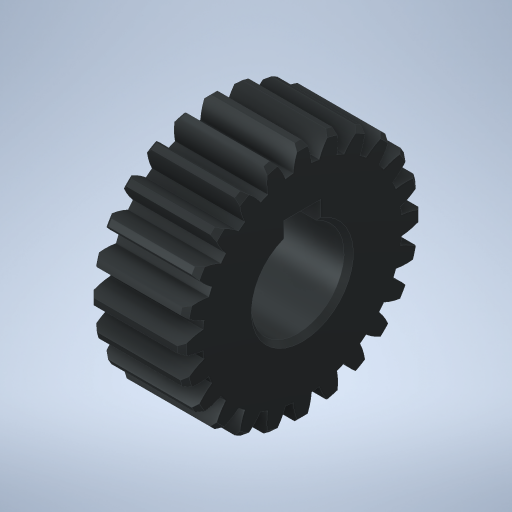
# Autodesk Inventor part: SSA1-24J10_On
Saved by Autodesk Inventor 2023 (Build 270158000, 158)
## iProperties
Category: PARTsolutions
Company: KHK
Created: 2023-07-21
Part Number: SSA1-24J10_On
Material: Iron, Cast
Catalog Web Link: www.cadenas.de
Description: Steel, Hubless Spur Gears (SSA)-
Vendor: KHK
Document SubType Name: Modeling
Designer: psAdmin
Manufacturer: KHK
Mass: 25.4574 g
Surface Area: 25.5099 cm^2
Volume: 3.56048 cm^3
Density: 7.15 g/cm^3
Appearance: Iron Gray
PSOL_IDENT_0: {$CADENAS_DATA/23d-libs/khk/spur_gears/steel_hubless_spur_gears_ssa.prj},198 {VTYP=3D},{NB=SSA1-24J1
PSOL_IDENT_1: 0_On},{LINA=SSA1-24J10},{NN=Steel, Hubless Spur Gears (SSA)},{DATE=06.10.2022 23:14:57},{GEOMDATE=26
PSOL_IDENT_2: .04.2021 06:49:50},{VERSION=},{LINEID=1180},{WBVAR=TOOTH,HT},{WBNUMERIC=}  {NB=SSA1-24J10_On},{LINA=
PSOL_IDENT_3: SSA1-24J10},{KT=DUMMY},{CN=SSA1-24J10},{CN1=SSA1-24J10},{A=10},{VER=1},{KW=4},{KD=1.8},{S=S5K},{SOLD=
PSOL_IDENT_4: S5K},{M=1},{MX=1.000},{Z=24},{B=0},{C=24.0},{D=26.0},{E=10},{F=0},{H=0},{I=0},{WMF=S5001.WMF},{N=0.5
PSOL_IDENT_5: },{L=0.5},{R=0},{L2=0},{VERS=0},{TOOTH=On},{HT=}
NB: SSA1-24J10_On
NN: Steel, Hubless Spur Gears (SSA)
NBSYN: $CN._$TOOTH.
LINA: SSA1-24J10
CATALOG: KHK
CN: SSA1-24J10
A: 10
KW: 4
KD: 1.8
S: S5K
M: 1
Z: 24
C: 24
D: 26
E: 10
TOOTH: On
HT: without
SUPPLIER: KHK
ARTICLENO: SSA1-24J10_On
BOMINFO: SSA1-24J10
CREATOR: CADENAS GmbH
Title: SSA1-24J10
Author: Cadenas PARTsolutions
Autodesk Inventor part; units mm, degrees
ref_plane "YZ Plane" through (0, 0, 0) normal (1, 0, 0) x (0, 1, 0)
ref_plane "XZ Plane" through (0, 0, 0) normal (0, 1, 0) x (-1, 0, 0)
ref_plane "XY Plane" through (0, 0, 0) normal (0, 0, 1) x (1, 0, 0)
sketch "Sketch_1" plane through (0, 0, 0) normal (0, 0, 1) x (1, 0, 0)
  line L0 (10, 0) -> (0, 0)
  line L1 (0, 5.5) -> (0.5, 5)
  line L2 (0.5, 5) -> (9.5, 5)
  line L3 (9.5, 5) -> (10, 5.5)
  line L4 (10, 5.5) -> (10, 12.5)
  line L5 (10, 12.5) -> (9.5, 13)
  line L6 (9.5, 13) -> (0.5, 13)
  line L7 (0.5, 13) -> (0, 12.5)
  line L8 (0, 12.5) -> (0, 5.5)
  constraints: 18 end point
revolve "Revolution1" add sketch "Sketch_1" angle 360 about axis through (10, 0, 0) along (1, 0, 0)
sketch "Sketch_6" plane through (0, 0, 0) normal (1, 0, 0) x (0, 1, 0)
  line L0 (0, 2) -> (0, -2)
  line L1 (0, -2) -> (6.8, -2)
  line L2 (6.8, -2) -> (6.8, 2)
  line L3 (6.8, 2) -> (0, 2)
  constraints: 8 end point
extrude "Extrusion1" cut sketch "Sketch_6" along normal blind 10
sketch "Sketch_7" plane through (0, 0, 0) normal (1, 0, 0) x (0, 1, 0)
  line L0 (26, 26) -> (-26, 26)
  line L1 (-26, 26) -> (-26, -26)
  line L2 (-26, -26) -> (26, -26)
  line L3 (26, -26) -> (26, 26)
  arc A0 (0.3403, 12.9955) -> (-0.3403, 12.9955) centre (0, 0) ccw
  arc A1 (-0.3403, 12.9955) -> (-0.9836, 10.7049) centre (4.9998, 10.2601) ccw
  arc A2 (-0.9836, 10.7049) -> (-1.8205, 10.5947) centre (0, 0) ccw
  arc A3 (-1.8205, 10.5947) -> (-3.0348, 12.6408) centre (-7.485, 8.6164) ccw
  arc A4 (-3.0348, 12.6408) -> (-3.6922, 12.4647) centre (0, 0) ccw
  arc A5 (-3.6922, 12.4647) -> (-3.7208, 10.0856) centre (2.174, 11.2045) ccw
  arc A6 (-3.7208, 10.0856) -> (-4.5006, 9.7625) centre (0, 0) ccw
  arc A7 (-4.5006, 9.7625) -> (-6.2031, 11.4246) centre (-9.46, 6.3856) ccw
  arc A8 (-6.2031, 11.4246) -> (-6.7925, 11.0843) centre (0, 0) ccw
  arc A9 (-6.7925, 11.0843) -> (-6.2043, 8.7789) centre (-0.8, 11.3854) ccw
  arc A10 (-6.2043, 8.7789) -> (-6.874, 8.265) centre (0, 0) ccw
  arc A11 (-6.874, 8.265) -> (-8.9486, 9.4299) centre (-10.7904, 3.7195) ccw
  arc A12 (-8.9486, 9.4299) -> (-9.4299, 8.9486) centre (0, 0) ccw
  arc A13 (-9.4299, 8.9486) -> (-8.265, 6.874) centre (-3.7195, 10.7904) ccw
  arc A14 (-8.265, 6.874) -> (-8.7789, 6.2043) centre (0, 0) ccw
  arc A15 (-8.7789, 6.2043) -> (-11.0843, 6.7925) centre (-11.3854, 0.8) ccw
  arc A16 (-11.0843, 6.7925) -> (-11.4246, 6.2031) centre (0, 0) ccw
  arc A17 (-11.4246, 6.2031) -> (-9.7625, 4.5006) centre (-6.3856, 9.46) ccw
  arc A18 (-9.7625, 4.5006) -> (-10.0856, 3.7208) centre (0, 0) ccw
  arc A19 (-10.0856, 3.7208) -> (-12.4647, 3.6922) centre (-11.2045, -2.174) ccw
  arc A20 (-12.4647, 3.6922) -> (-12.6408, 3.0348) centre (0, 0) ccw
  arc A21 (-12.6408, 3.0348) -> (-10.5947, 1.8205) centre (-8.6164, 7.485) ccw
  arc A22 (-10.5947, 1.8205) -> (-10.7049, 0.9836) centre (0, 0) ccw
  arc A23 (-10.7049, 0.9836) -> (-12.9955, 0.3403) centre (-10.2601, -4.9998) ccw
  arc A24 (-12.9955, 0.3403) -> (-12.9955, -0.3403) centre (0, 0) ccw
  arc A25 (-12.9955, -0.3403) -> (-10.7049, -0.9836) centre (-10.2601, 4.9998) ccw
  arc A26 (-10.7049, -0.9836) -> (-10.5947, -1.8205) centre (0, 0) ccw
  arc A27 (-10.5947, -1.8205) -> (-12.6408, -3.0348) centre (-8.6164, -7.485) ccw
  arc A28 (-12.6408, -3.0348) -> (-12.4647, -3.6922) centre (0, 0) ccw
  arc A29 (-12.4647, -3.6922) -> (-10.0856, -3.7208) centre (-11.2045, 2.174) ccw
  arc A30 (-10.0856, -3.7208) -> (-9.7625, -4.5006) centre (0, 0) ccw
  arc A31 (-9.7625, -4.5006) -> (-11.4246, -6.2031) centre (-6.3856, -9.46) ccw
  arc A32 (-11.4246, -6.2031) -> (-11.0843, -6.7925) centre (0, 0) ccw
  arc A33 (-11.0843, -6.7925) -> (-8.7789, -6.2043) centre (-11.3854, -0.8) ccw
  arc A34 (-8.7789, -6.2043) -> (-8.265, -6.874) centre (0, 0) ccw
  arc A35 (-8.265, -6.874) -> (-9.4299, -8.9486) centre (-3.7195, -10.7904) ccw
  arc A36 (-9.4299, -8.9486) -> (-8.9486, -9.4299) centre (0, 0) ccw
  arc A37 (-8.9486, -9.4299) -> (-6.874, -8.265) centre (-10.7904, -3.7195) ccw
  arc A38 (-6.874, -8.265) -> (-6.2043, -8.7789) centre (0, 0) ccw
  arc A39 (-6.2043, -8.7789) -> (-6.7925, -11.0843) centre (-0.8, -11.3854) ccw
  arc A40 (-6.7925, -11.0843) -> (-6.2031, -11.4246) centre (0, 0) ccw
  arc A41 (-6.2031, -11.4246) -> (-4.5006, -9.7625) centre (-9.46, -6.3856) ccw
  arc A42 (-4.5006, -9.7625) -> (-3.7208, -10.0856) centre (0, 0) ccw
  arc A43 (-3.7208, -10.0856) -> (-3.6922, -12.4647) centre (2.174, -11.2045) ccw
  arc A44 (-3.6922, -12.4647) -> (-3.0348, -12.6408) centre (0, 0) ccw
  arc A45 (-3.0348, -12.6408) -> (-1.8205, -10.5947) centre (-7.485, -8.6164) ccw
  arc A46 (-1.8205, -10.5947) -> (-0.9836, -10.7049) centre (0, 0) ccw
  arc A47 (-0.9836, -10.7049) -> (-0.3403, -12.9955) centre (4.9998, -10.2601) ccw
  arc A48 (-0.3403, -12.9955) -> (0.3403, -12.9955) centre (0, 0) ccw
  arc A49 (0.3403, -12.9955) -> (0.9836, -10.7049) centre (-4.9998, -10.2601) ccw
  arc A50 (0.9836, -10.7049) -> (1.8205, -10.5947) centre (0, 0) ccw
  arc A51 (1.8205, -10.5947) -> (3.0348, -12.6408) centre (7.485, -8.6164) ccw
  arc A52 (3.0348, -12.6408) -> (3.6922, -12.4647) centre (0, 0) ccw
  arc A53 (3.6922, -12.4647) -> (3.7208, -10.0856) centre (-2.174, -11.2045) ccw
  arc A54 (3.7208, -10.0856) -> (4.5006, -9.7625) centre (0, 0) ccw
  arc A55 (4.5006, -9.7625) -> (6.2031, -11.4246) centre (9.46, -6.3856) ccw
  arc A56 (6.2031, -11.4246) -> (6.7925, -11.0843) centre (0, 0) ccw
  arc A57 (6.7925, -11.0843) -> (6.2043, -8.7789) centre (0.8, -11.3854) ccw
  arc A58 (6.2043, -8.7789) -> (6.874, -8.265) centre (0, 0) ccw
  arc A59 (6.874, -8.265) -> (8.9486, -9.4299) centre (10.7904, -3.7195) ccw
  arc A60 (8.9486, -9.4299) -> (9.4299, -8.9486) centre (0, 0) ccw
  arc A61 (9.4299, -8.9486) -> (8.265, -6.874) centre (3.7195, -10.7904) ccw
  arc A62 (8.265, -6.874) -> (8.7789, -6.2043) centre (0, 0) ccw
  arc A63 (8.7789, -6.2043) -> (11.0843, -6.7925) centre (11.3854, -0.8) ccw
  arc A64 (11.0843, -6.7925) -> (11.4246, -6.2031) centre (0, 0) ccw
  arc A65 (11.4246, -6.2031) -> (9.7625, -4.5006) centre (6.3856, -9.46) ccw
  arc A66 (9.7625, -4.5006) -> (10.0856, -3.7208) centre (0, 0) ccw
  arc A67 (10.0856, -3.7208) -> (12.4647, -3.6922) centre (11.2045, 2.174) ccw
  arc A68 (12.4647, -3.6922) -> (12.6408, -3.0348) centre (0, 0) ccw
  arc A69 (12.6408, -3.0348) -> (10.5947, -1.8205) centre (8.6164, -7.485) ccw
  arc A70 (10.5947, -1.8205) -> (10.7049, -0.9836) centre (0, 0) ccw
  arc A71 (10.7049, -0.9836) -> (12.9955, -0.3403) centre (10.2601, 4.9998) ccw
  arc A72 (12.9955, -0.3403) -> (12.9955, 0.3403) centre (0, 0) ccw
  arc A73 (12.9955, 0.3403) -> (10.7049, 0.9836) centre (10.2601, -4.9998) ccw
  arc A74 (10.7049, 0.9836) -> (10.5947, 1.8205) centre (0, 0) ccw
  arc A75 (10.5947, 1.8205) -> (12.6408, 3.0348) centre (8.6164, 7.485) ccw
  arc A76 (12.6408, 3.0348) -> (12.4647, 3.6922) centre (0, 0) ccw
  arc A77 (12.4647, 3.6922) -> (10.0856, 3.7208) centre (11.2045, -2.174) ccw
  arc A78 (10.0856, 3.7208) -> (9.7625, 4.5006) centre (0, 0) ccw
  arc A79 (9.7625, 4.5006) -> (11.4246, 6.2031) centre (6.3856, 9.46) ccw
  arc A80 (11.4246, 6.2031) -> (11.0843, 6.7925) centre (0, 0) ccw
  arc A81 (11.0843, 6.7925) -> (8.7789, 6.2043) centre (11.3854, 0.8) ccw
  arc A82 (8.7789, 6.2043) -> (8.265, 6.874) centre (0, 0) ccw
  arc A83 (8.265, 6.874) -> (9.4299, 8.9486) centre (3.7195, 10.7904) ccw
  arc A84 (9.4299, 8.9486) -> (8.9486, 9.4299) centre (0, 0) ccw
  arc A85 (8.9486, 9.4299) -> (6.874, 8.265) centre (10.7904, 3.7195) ccw
  arc A86 (6.874, 8.265) -> (6.2043, 8.7789) centre (0, 0) ccw
  arc A87 (6.2043, 8.7789) -> (6.7925, 11.0843) centre (0.8, 11.3854) ccw
  arc A88 (6.7925, 11.0843) -> (6.2031, 11.4246) centre (0, 0) ccw
  arc A89 (6.2031, 11.4246) -> (4.5006, 9.7625) centre (9.46, 6.3856) ccw
  arc A90 (4.5006, 9.7625) -> (3.7208, 10.0856) centre (0, 0) ccw
  arc A91 (3.7208, 10.0856) -> (3.6922, 12.4647) centre (-2.174, 11.2045) ccw
  arc A92 (3.6922, 12.4647) -> (3.0348, 12.6408) centre (0, 0) ccw
  arc A93 (3.0348, 12.6408) -> (1.8205, 10.5947) centre (7.485, 8.6164) ccw
  arc A94 (1.8205, 10.5947) -> (0.9836, 10.7049) centre (0, 0) ccw
  arc A95 (0.9836, 10.7049) -> (0.3403, 12.9955) centre (-4.9998, 10.2601) ccw
  constraints: 192 point on circle, 96 centre point, 8 end point
extrude "Extrusion2" cut sketch "Sketch_7" along normal blind 10
body "Solid1"
